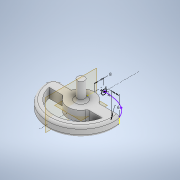
# Autodesk Inventor part: Servo_Kupplung_V3
Saved by Autodesk Inventor 2020 (Build 240168000, 168)
## iProperties
Created: 2020-09-04
Part Number: Servo_Kupplung_V3
Material: Generisch
Document SubType Name: Modeling
Designer: sp
Density: 1 g/cm^3
Appearance: Vorgabe
Author: sp
## iProperties of the stored document _3D-Druck.ipt
Created: 2020-09-04
Part Number: _3D-Druck
Material: Generisch
Document SubType Name: Modeling
Designer: sp
Density: 1 g/cm^3
Appearance: Vorgabe
Author: sp
Autodesk Inventor part; units mm, degrees
ref_plane "XZ Plane" through (0, 0, 0) normal (0, 1, 0) x (-1, 0, 0)
ref_plane "XY Plane" through (0, 0, 0) normal (0, 0, 1) x (1, 0, 0)
sketch "Skizze1" plane through (0, 0, 0) normal (0, 1, 0) x (-1, 0, 0)
  circle A0 centre (0, 0) radius 27.5
  circle A1 centre (0, 0) radius 22.5
  circle A2 centre (0, 0) radius 3.5
  line L0 (45.7225, 0) -> (-63.662, 0) construction
  line L1 (0, 78.2374) -> (0, -78.2374) construction
  circle A3 centre (15, 0) radius 2
  circle A4 centre (-15, 0) radius 2
  line L2 (0, 3.5) -> (15.1977, 1.9902)
  line L3 (15.1977, -1.9902) -> (0, -3.5)
  line L4 (-14.8023, -1.9902) -> (0, -3.5)
  line L5 (0, 3.5) -> (-15.1977, 1.9902)
  circle A5 centre (0, 0) radius 11
  line L6 (10.0387, 4.4973) -> (22.046, 4.4973)
  line L7 (-10.0387, 4.4973) -> (-22.046, 4.4973)
  line L8 (10.0387, -4.4973) -> (22.046, -4.4973)
  line L9 (-10.0387, -4.4973) -> (-22.046, -4.4973)
  point P0 (27.1298, 4.4973)
  point P1 (-27.023, -5.1)
  point P2 (13.75, -23.8157)
  point P3 (-13.75, 23.8157)
  point P4 (-0.6886, 3.4316)
  point P5 (0.6886, 3.4316)
  point P6 (0.6886, -3.4316)
  point P7 (-0.7066, -3.4279)
  dimension "d0" = 55
  dimension "d1" = 45
  dimension "d2" = 7
  dimension "d3" = 4
  dimension "d4" = 4
  dimension "d5" = 15
  dimension "d6" = 22
  constraints: 20 end point, 18 point on circle, 9 point on line, 6 centre point, 4 coincident, 3 horizontal, 2 midpoint, 1 parallel, 1 symmetric about line, 1 tangent, 1 vertical
  measures "d0" diameter of A0
  measures "d1" diameter of A1
  measures "d2" diameter of A2
  measures "d3" diameter of A3
  measures "d4" diameter of A4
  measures "d5" distance of point (0, 0) A3.centre
  measures "d6" diameter of A5
ref_plane "Arbeitsebene1" through (0, 3.7, 0) normal (0, 1, 0) x (1, 0, 0)
extrude "Extrusion3" add sketch "Skizze1" along normal blind 8 contours A0 | A1 L8 A5 L3 A3 L2 L6 | L7 A5 L5 A4 L4 L9 A1 | A5 L2 A2 L5 | A5 L4 A2 L3
sketch "Skizze3" plane through (0, 8, 0) normal (0, 1, 0) x (1, 0, 0)
  arc A0 (22.046, 4.4973) -> (-22.046, 4.4973) centre (0, 0) ccw projected
  arc A1 (-22.046, -4.4973) -> (22.046, -4.4973) centre (0, 0) ccw projected
  line L0 (-22.046, 4.4973) -> (22.046, 4.4973)
  line L1 (22.046, 4.4973) -> (22.046, -4.4973)
  line L2 (22.046, -4.4973) -> (-22.046, -4.4973)
  line L3 (-22.046, -4.4973) -> (-22.046, 4.4973)
  constraints: 8 end point, 2 parallel, 1 horizontal, 1 perpendicular, 1 point on circle
extrude "Extrusion4" add sketch "Skizze3" against normal blind 3 contours L1 L2 L3 L0
sketch "Skizze7" plane through (0, 8, 0) normal (0, 1, 0) x (1, 0, 0)
  arc A0 (22.046, 4.4973) -> (-22.046, 4.4973) centre (0, 0) ccw projected
  line L0 (-22.046, 4.4973) -> (-27.1298, 4.4973)
  circle A1 centre (0, 0) radius 27.5 projected
  line L1 (22.046, 4.4973) -> (10.0387, 4.4973) projected
  line L2 (22.046, 4.4973) -> (27.1412, 4.4973)
  line L3 (27.1412, 4.4973) -> (9.9712, 4.4973)
  arc A2 (10.0387, 4.4973) -> (-10.0387, 4.4973) centre (0, 0) ccw projected
  line L4 (-22.046, 4.4973) -> (-10.0387, 4.4973)
  circle A3 centre (0, 0) radius 11
  circle A4 centre (0, 0) radius 27.5
  point P0 (27.1298, 4.4973)
  constraints: 8 end point, 2 centre point, 2 coincident, 2 horizontal, 2 point on line, 3 other
extrude "Extrusion8" cut sketch "Skizze7" against normal blind 10 contours L1 A2 L4 A0 | A0 L0 A1 L2
fillet "Rundung8" radius 6 1 edges at (-27.1298, 4, -4.4973)
fillet "Rundung9" radius 2 6 edges at (-25.8358, 0, -2.589) (-15.743, 0, -4.4973) (3.2133, 0, 27.3116) (-25.8358, 8, -2.589) (-15.743, 8, -4.4973) (3.2133, 8, 27.3116)
sketch "Skizze9" plane through (0, 8, 0) normal (0, 1, 0) x (1, 0, 0)
  circle A0 centre (0, 0) radius 3
  dimension "d47" = 6
  constraints: 1 centre point, 1 coincident
  measures "d47" diameter of A0
extrude "Extrusion9" add sketch "Skizze9" along normal blind 15
fillet "Rundung10" radius 2 3 edges at (10.0387, 4, 4.4973) (10.0387, 4, -4.4973) (-10.0387, 4, 4.4973)
fillet "Rundung11" radius 2 1 edges at (-3, 8, 0)
ref_plane "Arbeitsebene4" through (0, 0, 0) normal (1, 0, 0) x (0, 1, 0)
sketch "Skizze10" plane through (27.1298, 2, -4.4973) normal (0, 0, -1) x (-1, 0, 0)
  line L0 (0, 0) -> (0, 4) projected
  line L1 (0, 2) -> (17.4598, 2)
  circle A0 centre (6, 2) radius 3
  point P0 (27.1298, -2)
  dimension "d53" = 6
  dimension "d54" = 6
  constraints: 2 end point, 1 centre point, 1 horizontal, 1 midpoint, 1 point on line
  measures "d53" diameter of A0
  measures "d54" horizontal distance of L0.end A0.centre
sketch "Skizze11" plane through (0, 0, 0) normal (1, 0, 0) x (0, 1, 0)
  line L0 (4, -48.7659) -> (4, 34.6929) construction
  line L1 (8, -11) -> (8, -2.4973) construction
  circle A0 centre (4, -19) radius 2
  point P0 (0, 0)
  point P1 (8, -5.4977)
  dimension "d55" = 4
  dimension "d56" = 4
  dimension "d57" = 8
  constraints: 2 end point, 1 centre point, 1 point on line, 1 vertical
  measures "d55" distance between parallel lines of L0 L1
  measures "d56" diameter of A0
  measures "d57" vertical distance of L1.start A0.centre
sketch "Skizze12" plane through (0, 3.7, 0) normal (0, 1, 0) x (1, 0, 0)
  arc A0 (-25.4376, -1.7823) -> (25.1003, 4.4973) centre (0, 0) ccw projected
  spline S0 degree 2 poles (25.1003, 4.4973) (21.7392, 19.3697) (0, 19.7453) knots 0 0 0 1 1 1
  point P0 (18.4599, 14.8701)
  constraints: 3 other
